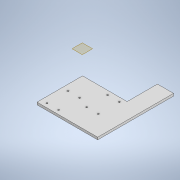
# Autodesk Inventor part: borard2_L
Saved by Autodesk Inventor 2020 (Build 240168000, 168)
## iProperties
Created: 2022-07-25
Part Number: borard2_L
Material: 일반
Document SubType Name: Modeling
Designer: SeungJin
Density: 1 g/cm^3
Appearance: 기본값
Author: SeungJin
Autodesk Inventor part; units mm, degrees
ref_plane "YZ Plane" through (0, 0, 0) normal (1, 0, 0) x (0, 1, 0)
ref_plane "XZ Plane" through (0, 0, 0) normal (0, 1, 0) x (-1, 0, 0)
ref_plane "XY Plane" through (0, 0, 0) normal (0, 0, 1) x (1, 0, 0)
ref_plane "작업 평면1" through (-145.5, 0, 75) normal (0, 1, 0) x (1, 0, 0)
sketch "스케치1" plane through (-145.5, 0, 75) normal (0, 1, 0) x (1, 0, 0)
  line L0 (0, -152.5) -> (185.5, -152.5)
  line L1 (185.5, -152.5) -> (185.5, 10)
  line L2 (185.5, 10) -> (75, 10)
  line L3 (75, 10) -> (75, 0)
  line L4 (75, 0) -> (0, 0)
  line L5 (0, 0) -> (0, -152.5)
  line L6 (185.5, 10) -> (75, 10)
  line L7 (185.5, -55) -> (185.5, 10)
  line L8 (195.5, 10) -> (195.5, -55)
  line L9 (0, 10) -> (151, 10)
  line L10 (151, 10) -> (151, -55)
  line L11 (151, -55) -> (0, -55)
  line L12 (0, -55) -> (0, 10)
  line L13 (55.5, -55) -> (55.5, -152.5)
  point P0 (151, 10)
  dimension "d4" = 10
  dimension "d41" = 151
  dimension "d42" = 65
  dimension "d43" = 130
  constraints: 28 end point, 2 parallel, 2 perpendicular, 2 point on line, 1 horizontal, 3 other
  measures "d4" distance between parallel lines of L8 L1
  measures "d41" distance of L10.end L11.end
  measures "d42" distance of L9.end L10.end
  measures "d43" distance between parallel lines of L1 L13
extrude "돌출1" add sketch "스케치1" along normal blind 5 contours L13 L11 L10 L2 L1 L0
sketch "스케치3" plane through (-145.5, 0, 75) normal (0, -1, 0) x (1, 0, 0)
  line L0 (55.5, 152.5) -> (185.5, 152.5) projected
  line L1 (55.5, 146.25) -> (105.5, 146.25)
  line L2 (105.5, 146.25) -> (105.5, 96.25)
  line L3 (105.5, 96.25) -> (55.5, 96.25)
  line L4 (55.5, 96.25) -> (55.5, 146.25)
  line L5 (155.5, 61.25) -> (105.5, 61.25)
  line L6 (105.5, 61.25) -> (105.5, 111.25)
  line L7 (105.5, 111.25) -> (155.5, 111.25)
  line L8 (155.5, 111.25) -> (155.5, 61.25)
  line L9 (68, 143.75) -> (93, 143.75)
  line L10 (93, 143.75) -> (93, 98.75)
  line L11 (93, 98.75) -> (68, 98.75)
  line L12 (68, 98.75) -> (68, 143.75)
  line L13 (118, 108.75) -> (143, 108.75)
  line L14 (143, 108.75) -> (143, 63.75)
  line L15 (143, 63.75) -> (118, 63.75)
  line L16 (118, 63.75) -> (118, 108.75)
  line L17 (55.5, 55) -> (55.5, 152.5) projected
  line L18 (151, 55) -> (55.5, 55) projected
  line L19 (151, -10) -> (151, 55) projected
  line L20 (185.5, -10) -> (151, -10) projected
  line L21 (185.5, 152.5) -> (185.5, -10) projected
  point P0 (145.5, -75)
  point P1 (130, 103.75)
  point P2 (134.5, 103.75)
  point P3 (68, 121.25)
  point P4 (55.5, 121.25)
  point P5 (118, 86.25)
  point P6 (105.5, 86.25)
  point P7 (130.5, 108.75)
  point P8 (130.5, 111.25)
  point P9 (80.5, 143.75)
  point P10 (80.5, 146.25)
  point P11 (80.5, 96.25)
  point P12 (80.5, 98.75)
  point P13 (130.5, 61.25)
  point P14 (130.5, 63.75)
  dimension "d32" = 50
  dimension "d34" = 50
  dimension "d35" = 25
  dimension "d36" = 45
  dimension "d37" = 25
  dimension "d38" = 45
  dimension "d39" = 50
  dimension "d40" = 50
  constraints: 32 end point, 12 midpoint, 8 coincident, 3 vertical alignment, 1 point on line
  measures "d32" distance of L2.end L3.end
  measures "d34" distance of L5.end L6.end
  measures "d35" distance of L10.end L11.end
  measures "d36" distance of L9.end L10.end
  measures "d37" distance of L14.end L15.end
  measures "d38" distance of L13.end L14.end
  measures "d39" distance between parallel lines of L3 L1
  measures "d40" distance between parallel lines of L6 L8
hole "구멍1" at (-77.5, 0, 218.75) at (-77.5, 0, 173.75) at (-52.5, 0, 218.75) at (-52.5, 0, 173.75) at (-27.5, 0, 183.75) at (-2.5, 0, 183.75) at (-2.5, 0, 138.75) at (-27.5, 0, 138.75) direction (0, 1, 0) diameter 3.4 end through all counterbore diameter 6 counterbore depth 3 clearance for "Hex Head Cap Screw ISO 24017" size "M3" standard "ISO"
